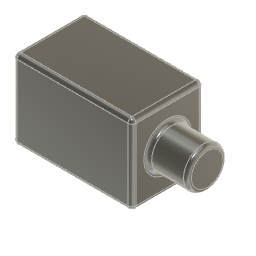
_Sign Holder, Top Hole.7aac6f4d-4736-4917-9fa4-9258fc648495 (Autodesk Fusion 360 design; units mm, degrees)
Autodesk Fusion 360 part; units mm, degrees
sketch "Sketch1" plane through (0, 0, 0) normal (0, 0, 1) x (1, 0, 0)
  line L0 (0, 0) -> (-38.1, 0)
  line L1 (-38.1, 0) -> (-38.1, -38.1)
  line L2 (-38.1, -38.1) -> (0, -38.1)
  line L3 (0, -38.1) -> (0, 0)
  dimension "d1" = 38.1
  dimension "d2" = 38.1
  constraint horizontal L0
  constraint vertical L1
  constraint horizontal L2
  constraint vertical L3
  constraint coincident L0.start L3.end
  measures "d1" distance of L0.start L0.end
  measures "d2" distance of L0.start L2.end
extrude "Extrude1" add sketch "Sketch1" along normal blind 25.4
sketch "Sketch2" plane through (0, 0, 0) normal (1, 0, 0) x (0, 1, 0)
  line L0 (-38.1, 0) -> (0, 0)
  line L1 (0, 0) -> (0, 25.4)
  line L2 (0, 25.4) -> (-38.1, 25.4)
  line L3 (-38.1, 25.4) -> (-38.1, 0)
  line L4 (-38.1, 0) -> (-19.05, 0)
  line L5 (-19.05, 0) -> (-19.05, 12.7)
  circle A0 centre (-19.05, 12.7) radius 6.35
  dimension "d5" = 12.7
  constraint coincident L0.start L3.end
  constraint midpoint L0 L4.end
  constraint perpendicular L4 L5
  constraint coincident L5.end A0.centre
  measures "d5" diameter of A0
extrude "Extrude2" add sketch "Sketch2" along normal blind 12.7 contours A0
sketch "Sketch3" plane through (0, 0, 0) normal (0, 0, -1) x (1, 0, 0)
  line L0 (0, 0) -> (0, 38.1)
  line L1 (0, 38.1) -> (-38.1, 38.1)
  line L2 (-38.1, 38.1) -> (-38.1, 0)
  line L3 (-38.1, 0) -> (0, 0)
  line L4 (-38.1, 19.05) -> (-25.4, 19.05)
  line L5 (0, 19.05) -> (-12.7, 19.05)
  circle A0 centre (-12.7, 19.05) radius 3.175
  circle A1 centre (-25.4, 19.05) radius 3.175
  dimension "d9" = 12.7
  dimension "d10" = 12.7
  dimension "d11" = 6.35
  dimension "d12" = 6.35
  constraint midpoint L2 L4.start
  constraint perpendicular L2 L4
  constraint midpoint L0 L5.start
  constraint perpendicular L0 L5
  constraint coincident L5.end A0.centre
  constraint coincident L4.end A1.centre
  measures "d9" distance of L4.start L4.end
  measures "d10" distance of L5.start L5.end
  measures "d11" diameter of A0
  measures "d12" diameter of A1
extrude "Extrude3" add sketch "Sketch3" along normal blind 5.08 contours A1
extrude "Extrude4" add sketch "Sketch3" along normal blind 5.08 contours A0
extrude "Extrude5" cut 1 faces at (-12.7, 0, 8.4667) along direction (0, -1, 0) blind 7.62
extrude "Extrude6" cut 1 faces at (-25.4, -38.1, 8.4667) along direction (0, 1, 0) blind 7.62
extrude "Extrude7" cut 2 faces at (-13.6995, -18.8958, -5.08) (-24.8413, -17.3109, -5.08) along direction (0, 0, 1) blind 2.54
fillet "Fillet1" radius 1.27 12 faces at (-25.4, -30.48, 8.4667) (0, -18.8918, 2.1226) (-38.1, -15.24, 8.4667) (12.7, -19.3851, 13.862) (-12.7, -7.62, 8.4667) (-12.7, -22.86, 25.4) (4.2333, -12.7079, 13.0165) (-34.925, -19.05, 0) (-13.6995, -18.8958, -2.54) (-24.8413, -17.3109, -2.54) (-9.5408, -18.7339, -0.8467) (-22.2408, -19.3661, -1.6933)
sketch "Sketch4" plane through (-38.1, 0, 0) normal (-1, 0, 0) x (0, -1, 0)
  line L0 (29.21, 1.27) -> (29.21, 24.13)
  line L1 (29.21, 24.13) -> (8.89, 24.13)
  line L2 (8.89, 24.13) -> (8.89, 1.27)
  line L3 (8.89, 1.27) -> (29.21, 1.27)
  circle A0 centre (19.05, 12.7) radius 6.35
  line L4 (19.05, 12.7) -> (19.05, 19.05)
  line L5 (18.542, 19.812) -> (19.558, 19.812)
  line L6 (19.558, 19.812) -> (19.558, 18.288)
  line L7 (19.558, 18.288) -> (18.542, 18.288)
  line L8 (18.542, 18.288) -> (18.542, 19.812)
  line L9 (18.542, 19.812) -> (19.558, 18.288) construction
  line L10 (19.558, 19.812) -> (18.542, 18.288) construction
  point P0 (19.05, 19.05)
  dimension "d29" = 1.016
  dimension "d30" = 1.524
  constraint coincident A0.centre L4.start
  constraint coincident A0 P0
  constraint vertical L4
  constraint horizontal L5
  constraint perpendicular L5 L6
  constraint parallel L5 L7
  constraint parallel L6 L8
  constraint coincident L9 P0
  constraint coincident L10 P0
  constraint coincident P0 L4.end
  measures "d29" distance of L6.end L7.end
  measures "d30" distance of L5.end L6.end
extrude "Extrude8" cut sketch "Sketch4" against normal blind 12.7 contours A0 L6 L7 L8 | A0 L4 L6 L7 | A0 L5 L6 L8 | A0 L4 L7 L8
fillet "Fillet2" radius 1.27 1 edges at (-38.1, -19.05, 6.35)
equation "d6 = ( 1 / 2 ) * 1 in"
